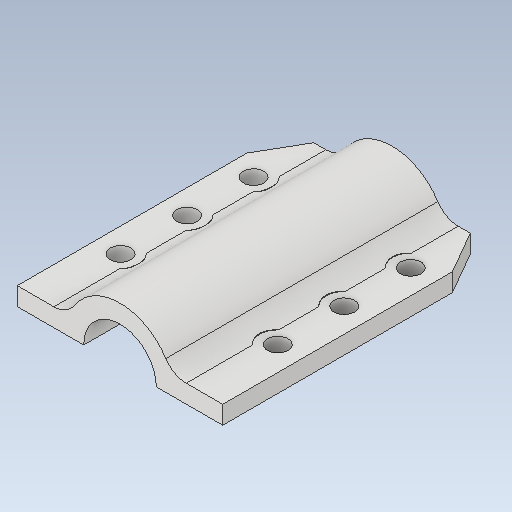
# Autodesk Inventor part: Cartesian1_X_RodCover
Saved by Autodesk Inventor 2020 (Build 240168000, 168)
## iProperties
Created: 2020-03-07
Part Number: Cartesian1_X_RodCover
Material: Tworzywo sztuczne ABS
Document SubType Name: Modeling
Designer: invin
Density: 1.06 g/cm^3
Appearance: Gładki — biały
Mass: 5.53412 g
Surface Area: 40.7862 cm^2
Volume: 5.22087 cm^3
Author: invin
Autodesk Inventor part; units mm, degrees
ref_plane "YZ Plane" through (0, 0, 0) normal (1, 0, 0) x (0, 1, 0)
ref_plane "XZ Plane" through (0, 0, 0) normal (0, 1, 0) x (-1, 0, 0)
sketch "Szkic1" plane through (0, 0, 0) normal (0, 0, 1) x (1, 0, 0)
  circle A0 centre (0, 0) radius 6
  circle A1 centre (0, 0) radius 9
  dimension "d0" = 12
  dimension "d1" = 18
  constraints: 2 centre point, 2 coincident
  measures "d0" diameter of A0
  measures "d1" diameter of A1
extrude "Wyciągnięcie proste1" add sketch "Szkic1" along normal blind 50
sketch "Szkic2" plane through (0, 0, 50) normal (0, 0, 1) x (1, 0, 0)
  line L0 (-7.2, 0) -> (-20, 0)
  line L1 (-20, 0) -> (-20, 3)
  line L2 (-20, 3) -> (-7.2, 3)
  line L3 (-7.2, 3) -> (-7.2, 0)
  point P0 (0, 0)
  dimension "d4" = 3
  dimension "d5" = 7.2
  dimension "d6" = 20
  constraints: 8 end point, 2 parallel, 1 horizontal, 1 perpendicular
  measures "d4" distance between parallel lines of L0 L2
  measures "d5" distance from line of point (0, 0) L3
  measures "d6" distance from line of L1 point (0, 0)
extrude "Wyciągnięcie proste2" add sketch "Szkic2" against normal blind 50
ref_plane "Płaszczyzna konstrukcyjna1" through (0, 0, 50) normal (-1, 0, 0) x (0, 0, 1)
sketch "Szkic3" plane through (0, 0, 50) normal (0, 0, 1) x (1, 0, 0)
  arc A0 (-9, 0) -> (-8.4853, 3) centre (0, 0) ccw projected
  line L0 (-9, 0) -> (13.5216, 0)
  line L1 (13.5216, 0) -> (13.5216, -10.7801)
  line L2 (13.5216, -10.7801) -> (-9, -10.7801)
  line L3 (-9, -10.7801) -> (-9, 0)
  constraints: 8 end point, 2 parallel, 1 horizontal, 1 perpendicular
extrude "Wyciągnięcie proste3" cut sketch "Szkic3" against normal blind 50
sketch "Szkic5" plane through (-20, 3, 50) normal (0, 1, 0) x (1, 0, 0)
  circle A0 centre (7, 13.1) radius 1.7
  circle A1 centre (7, 24.1) radius 1.7
  circle A2 centre (7, 35.1) radius 1.7
  line L0 (0, 0) -> (11.5147, 0) projected
  line L1 (20, -10) -> (20, 60) projected
  point P0 (20, 50)
  dimension "d12" = 3.4
  dimension "d13" = 3.4
  dimension "d14" = 3.4
  dimension "d16" = 13.1
  dimension "d17" = 11
  dimension "d18" = 11
  dimension "d19" = 13
  dimension "d20" = 0
  dimension "d21" = 0
  constraints: 3 centre point
  measures "d12" diameter of A0
  measures "d13" diameter of A1
  measures "d14" diameter of A2
  measures "d16" distance from line of L0 A0.centre
  measures "d17" distance of A0.centre A1.centre
  measures "d18" distance of A2.centre A1.centre
  measures "d19" distance from line of L1 A2.centre
  measures "d20" horizontal distance of A2.centre A1.centre
  measures "d21" horizontal distance of A1.centre A0.centre
extrude "Wyciągnięcie proste4" cut sketch "Szkic5" against normal blind 50
fillet "Zaokrąglenie1" radius 4 1 edges at (-8.4853, 3, 25)
mirror "Odbij1" about plane through (0, 0, 50) normal (-1, 0, 0) of "Wyciągnięcie proste2", "Wyciągnięcie proste4", "Zaokrąglenie1"
sketch "Szkic6" plane through (6, 0, 0) normal (0, -1, 0) x (1, 0, 0)
  line L0 (15.0838, 0) -> (-24.5144, 0)
  line L1 (-24.5144, 0) -> (-24.5144, 5)
  line L2 (-24.5144, 5) -> (15.0838, 5)
  line L3 (15.0838, 5) -> (15.0838, 0)
  point P0 (-6, 0)
  dimension "d28" = 5
  constraints: 8 end point, 2 parallel, 1 horizontal, 1 perpendicular
  measures "d28" distance between parallel lines of L0 L2
extrude "Wyciągnięcie proste5" cut sketch "Szkic6" against normal blind 50
sketch "Szkic8" plane through (-20, 3, 50) normal (0, 1, 0) x (1, 0, 0)
  line L0 (-3.2921, -2.8939) -> (3, -2.8939)
  line L1 (3, -2.8939) -> (3, 49.96)
  line L2 (3, 49.96) -> (-3.2921, 49.96)
  line L3 (-3.2921, 49.96) -> (-3.2921, -2.8939)
  line L4 (37, 48) -> (48.6867, 48)
  line L5 (48.6867, 48) -> (48.6867, -7.6985)
  line L6 (48.6867, -7.6985) -> (37, -7.6985)
  line L7 (37, -7.6985) -> (37, 48)
  circle A0 centre (33, 35.1) radius 1.7 projected
  circle A1 centre (7, 35.1) radius 1.7 projected
  point P0 (20, 50)
  dimension "d32" = 4
  dimension "d33" = 4
  constraints: 16 end point, 4 parallel, 2 horizontal, 2 perpendicular
  measures "d32" distance from line of L7 A0.centre
  measures "d33" distance from line of A1.centre L1
extrude "Wyciągnięcie proste6" cut sketch "Szkic8" against normal blind 50 contours L3 L2 L1 L0 | L4 L5 L6 L7
chamfer "Faza2" distance 7 angle 30 1 edges at (17, 1.5, 5) measured on face at (17, 1, 35)
chamfer "Faza3" distance 7 angle 30 1 edges at (-17, 1.5, 5) measured on face at (-17, 1, 35)
sketch "Szkic9" plane through (-20, 3, 0.04) normal (0, 0, 1) x (1, 0, 0)
  line L0 (-2.5115, 2.374) -> (2.3445, 2.374)
  line L1 (2.3445, 2.374) -> (2.3445, -9.0767)
  line L2 (2.3445, -9.0767) -> (-2.5115, -9.0767)
  line L3 (-2.5115, -9.0767) -> (-2.5115, 2.374)
  point P0 (20, -3)
  constraints: 8 end point, 2 parallel, 1 horizontal, 1 perpendicular
extrude "Wyciągnięcie proste7" cut sketch "Szkic9" against normal blind 50
sketch "Szkic11" plane through (-10.9545, 3, 50) normal (0, 1, 0) x (1, 0, 0)
  circle A0 centre (-2.0455, 35.1) radius 3
  circle A1 centre (-2.0455, 13.1) radius 3
  circle A2 centre (-2.0455, 24.1) radius 3
  circle A3 centre (23.9545, 35.1) radius 3
  circle A4 centre (23.9545, 24.1) radius 3
  circle A5 centre (23.9545, 13.1) radius 3
  circle A6 centre (23.9545, 35.1) radius 1.7 projected
  circle A7 centre (23.9545, 24.1) radius 1.7 projected
  circle A8 centre (23.9545, 13.1) radius 1.7 projected
  circle A9 centre (-2.0455, 13.1) radius 1.7 projected
  circle A10 centre (-2.0455, 24.1) radius 1.7 projected
  circle A11 centre (-2.0455, 35.1) radius 1.7 projected
  point P0 (10.9545, 50)
  dimension "d47" = 6
  dimension "d48" = 6
  dimension "d49" = 6
  dimension "d50" = 6
  dimension "d51" = 6
  dimension "d52" = 6
  constraints: 6 centre point, 6 concentric
  measures "d47" diameter of A0
  measures "d48" diameter of A1
  measures "d49" diameter of A2
  measures "d50" diameter of A3
  measures "d51" diameter of A4
  measures "d52" diameter of A5
extrude "Wyciągnięcie proste9" cut sketch "Szkic11" along normal blind 50
